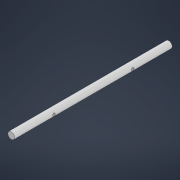
# Autodesk Inventor part: Eixo_traseiro
Saved by Autodesk Inventor 2022 (Build 260153000, 153)
## iProperties
Created: 2022-06-10
Part Number: Eixo_traseiro
Material: Generic
Document SubType Name: Modeling
Designer: Gugarauj07
Density: 1 g/cm^3
Appearance: Default
Author: Gugarauj07
Autodesk Inventor part; units mm, degrees
ref_plane "YZ Plane" through (0, 0, 0) normal (1, 0, 0) x (0, 1, 0)
ref_plane "XZ Plane" through (0, 0, 0) normal (0, 1, 0) x (-1, 0, 0)
ref_plane "XY Plane" through (0, 0, 0) normal (0, 0, 1) x (1, 0, 0)
sketch "Sketch1" plane through (0, 0, 0) normal (1, 0, 0) x (0, 1, 0)
  line L0 (12.7, 300) -> (-12.7, 300)
  line L1 (-12.7, 300) -> (-12.7, -300)
  line L2 (-12.7, -300) -> (12.7, -300)
  line L3 (12.7, -300) -> (12.7, 300)
  line L4 (12.7, 300) -> (-12.7, -300) construction
  line L5 (-12.7, 300) -> (12.7, -300) construction
  circle A0 centre (0, 150) radius 5
  circle A1 centre (0, -150) radius 5
  line L6 (0, 0) -> (0, -150)
  dimension "d0" = 25.4
  dimension "d1" = 600
  dimension "d3" = 10
  dimension "d8" = 150
  constraints: 14 end point, 2 centre point, 2 midpoint, 2 parallel, 1 horizontal, 1 perpendicular, 1 vertical
  measures "d0" distance of L2.end L1.end
  measures "d1" distance of L0.end L1.end
  measures "d3" diameter of A0
  measures "d8" distance of L6.start L6.end
extrude "Extrusion1" add sketch "Sketch1" along normal blind 25.4
fillet "Fillet1" radius 12.7 4 edges at (25.4, -12.7, 0) (0, -12.7, 0) (25.4, 12.7, 0) (0, 12.7, 0)
body "Solid1"
